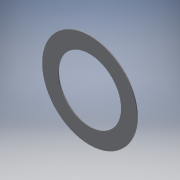
# Autodesk Inventor part: support ring
Saved by Autodesk Inventor 2017 (Build 210142000, 142)
## iProperties
Created: 2016-10-09
Part Number: support ring
Material: Aluminum 6061
Document SubType Name: Modeling
Designer: gus
Density: 2.7 g/cm^3
Appearance: Aluminum - Flat
Author: gus
Autodesk Inventor part; units mm, degrees
ref_plane "YZ Plane" through (0, 0, 0) normal (1, 0, 0) x (0, 1, 0)
ref_plane "XZ Plane" through (0, 0, 0) normal (0, 1, 0) x (-1, 0, 0)
ref_plane "XY Plane" through (0, 0, 0) normal (0, 0, 1) x (1, 0, 0)
sketch "Sketch1" plane through (0, 0, 0) normal (0, 0, 1) x (1, 0, 0)
  circle A0 centre (0, 0) radius 139.7
  circle A1 centre (0, 0) radius 88.9
  dimension "d0" = 279.4
  dimension "d1" = 50.8
  constraints: 2 centre point, 2 coincident
  measures "d0" diameter of A0
  measures "d1" radial gap between concentric circles of A0 A1
extrude "Extrusion1" add sketch "Sketch1" along normal blind 3.175
sketch "Sketch2" plane through (0, 0, 3.175) normal (0, 0, 1) x (1, 0, 0)
  circle A0 centre (0, 0) radius 120.2563 construction
  circle A1 centre (0, -120.2563) radius 2.5781
  circle A2 centre (120.2563, 0) radius 2.5781
  circle A3 centre (0, 120.2563) radius 2.5781
  circle A4 centre (-120.2563, 0) radius 2.5781
  line L0 (-120.2563, 0) -> (120.2563, 0) construction
  line L1 (0, -120.2563) -> (0, 120.2563) construction
  dimension "d4" = 240.5126
  dimension "d5" = 5.1562
  constraints: 5 centre point, 4 end point, 4 midpoint, 4 point on circle, 3 equal radius, 1 coincident, 1 horizontal, 1 perpendicular
  measures "d4" diameter of A0
  measures "d5" diameter of A1
extrude "Extrusion2" cut sketch "Sketch2" against normal blind 3.175
body "Solid1"
